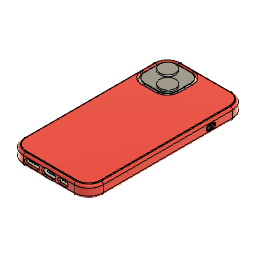
Day 10 - Phone Case v1 (Autodesk Fusion 360 design; units mm, degrees)
Autodesk Fusion 360 part; units mm, degrees
sketch "Sketch1" plane through (0, 0, 0) normal (0, 0, 1) x (1, 0, 0)
  line L0 (-24.135, 73.4) -> (24.135, 73.4)
  line L1 (35.8, 61.735) -> (35.8, -61.735)
  line L2 (24.135, -73.4) -> (-24.135, -73.4)
  line L3 (-35.8, -61.735) -> (-35.8, 61.735)
  arc A0 (-24.135, 73.4) -> (-35.8, 61.735) centre (-24.135, 61.735) ccw
  arc A1 (35.8, 61.735) -> (24.135, 73.4) centre (24.135, 61.735) ccw
  arc A2 (24.135, -73.4) -> (35.8, -61.735) centre (24.135, -61.735) ccw
  arc A3 (-35.8, -61.735) -> (-24.135, -73.4) centre (-24.135, -61.735) ccw
  point P0 (35.8, 73.4)
  point P1 (35.8, -73.4)
  point P2 (-35.8, -73.4)
  dimension "d1" = 71.6
  dimension "d2" = 146.8
  dimension "d3" = 11.665
  constraint horizontal L0
  constraint perpendicular L0 L1
  constraint parallel L0 L2
  constraint parallel L1 L3
  constraint tangent L0 A0
  constraint tangent L3 A0
  constraint coincident P0 L0
  constraint coincident P0 L1
  constraint tangent L0 A1
  constraint tangent L1 A1
  constraint equal A0 A1
  constraint coincident P1 L1
  constraint coincident P1 L2
  constraint tangent L1 A2
  constraint tangent L2 A2
  constraint equal A0 A2
  constraint coincident P2 L2
  constraint coincident P2 L3
  constraint tangent L2 A3
  constraint tangent L3 A3
  constraint equal A0 A3
  measures "d1" distance of P1 P2
  measures "d2" distance of P0 P1
  measures "d3" radius of A0
extrude "Extrude1" add sketch "Sketch1" along normal blind 7.8 makes body 1
fillet "Fillet1" radius 0.4 2 faces at (-11.9333, 20.5783, 7.8) (-11.9333, 20.5783, 0) on bodies 1
sketch "Sketch2" plane through (0, 0, 7.8) normal (0, 0, 1) x (-1, 0, 0)
  arc A0 (24.135, -73) -> (35.4, -61.735) centre (24.135, -61.735) ccw
  line L0 (35.4, -61.735) -> (35.4, 61.735)
  arc A1 (35.4, 61.735) -> (24.135, 73) centre (24.135, 61.735) ccw
  line L1 (24.135, 73) -> (-24.135, 73)
  arc A2 (-24.135, 73) -> (-35.4, 61.735) centre (-24.135, 61.735) ccw
  line L2 (-35.4, 61.735) -> (-35.4, -61.735)
  arc A3 (-35.4, -61.735) -> (-24.135, -73) centre (-24.135, -61.735) ccw
  line L3 (-24.135, -73) -> (24.135, -73)
  arc A4 (24.135, -73.4) -> (35.8, -61.735) centre (24.135, -61.735) ccw
  line L4 (35.8, 61.735) -> (35.8, -61.735)
  arc A5 (35.8, 61.735) -> (24.135, 73.4) centre (24.135, 61.735) ccw
  line L5 (-24.135, 73.4) -> (24.135, 73.4)
  arc A6 (-24.135, 73.4) -> (-35.8, 61.735) centre (-24.135, 61.735) ccw
  line L6 (-35.8, -61.735) -> (-35.8, 61.735)
  arc A7 (-35.8, -61.735) -> (-24.135, -73.4) centre (-24.135, -61.735) ccw
  line L7 (24.135, -73.4) -> (-24.135, -73.4)
  line L8 (21.4109, -73.4) -> (21.4109, -70.7)
  line L9 (35.8, -59.3465) -> (33.1, -59.3465)
  line L10 (24.118, -70.7) -> (11.082, -70.7)
  line L11 (2.1, -61.718) -> (2.1, -48.682)
  line L12 (11.082, -39.7) -> (24.118, -39.7)
  line L13 (33.1, -48.682) -> (33.1, -61.718)
  arc A8 (24.118, -70.7) -> (33.1, -61.718) centre (24.118, -61.718) ccw
  arc A9 (2.1, -61.718) -> (11.082, -70.7) centre (11.082, -61.718) ccw
  arc A10 (11.082, -39.7) -> (2.1, -48.682) centre (11.082, -48.682) ccw
  arc A11 (33.1, -48.682) -> (24.118, -39.7) centre (24.118, -48.682) ccw
  point P0 (33.1, -70.7)
  point P1 (2.1, -70.7)
  point P2 (33.1, -39.7)
  dimension "d8" = 2.7
  dimension "d9" = 2.7
  dimension "d10" = 31
  dimension "d11" = 31
  dimension "d12" = 8.982
  constraint coincident L7 L8.start
  constraint perpendicular L3 L8
  constraint coincident L4 L9.start
  constraint perpendicular L0 L9
  constraint horizontal L10
  constraint vertical L11
  constraint horizontal L12
  constraint vertical L13
  constraint coincident P0 L10
  constraint coincident P0 L13
  constraint tangent L10 A8
  constraint tangent L13 A8
  constraint coincident P1 L10
  constraint coincident P1 L11
  constraint tangent L10 A9
  constraint tangent L11 A9
  constraint equal A8 A9
  constraint tangent L11 A10
  constraint tangent L12 A10
  constraint equal A8 A10
  constraint coincident P2 L12
  constraint coincident P2 L13
  constraint tangent L12 A11
  constraint tangent L13 A11
  constraint equal A8 A11
  measures "d8" distance of L8.start L8.end
  measures "d9" distance of L9.start L9.end
  measures "d10" distance of P0 P1
  measures "d11" distance of P0 P2
  measures "d12" radius of A8
extrude "Extrude2" add sketch "Sketch2" along normal blind 2 contours L10 L11 L12 L13 A8 A9 A10 A11 bodies 1
fillet "Fillet2" radius 1.5 8 edges at (-33.1, 55.2, 7.8) (-30.4692, 68.0692, 7.8) (-17.6, 70.7, 7.8) (-4.7308, 68.0692, 7.8) (-2.1, 55.2, 7.8) (-4.7308, 42.3308, 7.8) (-17.6, 39.7, 7.8) (-30.4692, 42.3308, 7.8) on bodies 1
sketch "Sketch3" plane through (0, 0, 9.8) normal (0, 0, 1) x (-1, 0, 0)
  arc A0 (24.118, -70.7) -> (33.1, -61.718) centre (24.118, -61.718) ccw
  line L0 (33.1, -61.718) -> (33.1, -48.682)
  arc A1 (33.1, -48.682) -> (24.118, -39.7) centre (24.118, -48.682) ccw
  line L1 (24.118, -39.7) -> (11.082, -39.7)
  arc A2 (11.082, -39.7) -> (2.1, -48.682) centre (11.082, -48.682) ccw
  line L2 (2.1, -48.682) -> (2.1, -61.718)
  arc A3 (2.1, -61.718) -> (11.082, -70.7) centre (11.082, -61.718) ccw
  line L3 (11.082, -70.7) -> (24.118, -70.7)
  line L4 (21.9339, -70.7) -> (21.9339, -68.7)
  line L5 (33.1, -60.9415) -> (31.1, -60.9415)
  line L6 (12.075, -70.7) -> (12.075, -56.2)
  line L7 (33.1, -49.3388) -> (18.6, -49.3388)
  line L8 (31.1, -68.7) -> (23.6, -68.7)
  line L9 (31.1, -68.7) -> (31.1, -61.2)
  circle A4 centre (23.6, -61.2) radius 7.5
  line L10 (18.6, -56.2) -> (11.1, -56.2)
  line L11 (18.6, -56.2) -> (18.6, -48.7)
  circle A5 centre (11.082, -48.682) radius 7.518
  dimension "d17" = 2
  dimension "d18" = 2
  dimension "d19" = 14.5
  dimension "d20" = 14.5
  dimension "d21" = 7.5
  dimension "d22" = 7.5
  dimension "d23" = 7.5
  dimension "d24" = 7.5
  constraint coincident L3 L4.start
  constraint perpendicular L3 L4
  constraint coincident L0 L5.start
  constraint perpendicular L0 L5
  constraint coincident L3 L6.start
  constraint perpendicular L3 L6
  constraint coincident L0 L7.start
  constraint perpendicular L0 L7
  constraint parallel L3 L8
  constraint perpendicular L5 L9
  constraint coincident L8.end A4
  constraint tangent L8 A4
  constraint perpendicular L6 L10
  constraint perpendicular L7 L11
  constraint concentric A2 A5
  constraint coincident L11.end A5
  measures "d17" distance of L4.start L4.end
  measures "d18" distance of L5.start L5.end
  measures "d19" distance of L6.start L6.end
  measures "d20" distance of L7.start L7.end
  measures "d21" distance of L8.start L8.end
  measures "d22" distance of L8.start L9.end
  measures "d23" distance of L10.start L10.end
  measures "d24" distance of L10.start L11.end
extrude "Extrude3" add sketch "Sketch3" along normal blind 1.5 contours A4 L10 L11 | A5 picked at (25.4599, -63.0599) bodies 1
delete_face "DeleteFace1" 2 faces at (-18.4033, 56.2, 10.3) (-18.6, 56.0033, 10.3) on bodies 1
sketch "Sketch4" plane through (35.8, 0, 0) normal (1, 0, 0) x (0, 1, 0)
  line L0 (-61.735, 0.4) -> (61.735, 0.4)
  line L1 (61.735, 0.4) -> (61.735, 7.4)
  line L2 (61.735, 7.4) -> (-61.735, 7.4)
  line L3 (-61.735, 7.4) -> (-61.735, 0.4)
  line L4 (68.7, 11.3) -> (53.7, 11.3)
  line L5 (70.7, 9.8) -> (68.7, 9.8)
  line L6 (41.164, 9.8) -> (39.7, 9.8)
  line L7 (53.7, 11.3) -> (41.164, 11.3)
  arc A0 (70.7, 9.3) -> (72.2, 7.8) centre (72.2, 9.3) ccw
  arc A1 (38.2, 7.8) -> (39.7, 9.3) centre (38.2, 9.3) ccw
  line L8 (70.7, 9.3) -> (70.7, 9.8)
  line L9 (72.2, 7.8) -> (73, 7.8)
  line L10 (-61.735, 7.8) -> (38.2, 7.8)
  line L11 (-73, 7.8) -> (-61.735, 7.8)
  line L12 (39.7, 9.3) -> (39.7, 9.8)
  arc A2 (73, 0) -> (73.4, 0.4) centre (73, 0.4) ccw
  line L13 (73, 0) -> (61.735, 0)
  line L14 (61.735, 0) -> (-61.735, 0)
  arc A3 (-73.4, 0.4) -> (-73, 0) centre (-73, 0.4) ccw
  line L15 (-61.735, 0) -> (-73, 0)
  line L16 (73.4, 0.4) -> (73.4, 7.4)
  arc A4 (73.4, 7.4) -> (73, 7.8) centre (73, 7.4) ccw
  arc A5 (-73, 7.8) -> (-73.4, 7.4) centre (-73, 7.4) ccw
  line L17 (-73.4, 0.4) -> (-73.4, 7.4)
  line L18 (41.164, 9.8) -> (41.164, 11.3)
  line L19 (68.7, 9.8) -> (68.7, 11.3)
  line L20 (73.4, 3.9) -> (44.07, 3.9)
  line L21 (44.07, 3.9) -> (41.27, 3.9)
  line L22 (43.5325, 4.975) -> (39.0075, 4.975)
  line L23 (38.47, 4.4375) -> (38.47, 3.3625)
  line L24 (39.0075, 2.825) -> (43.5325, 2.825)
  line L25 (44.07, 3.3625) -> (44.07, 4.4375)
  arc A6 (44.07, 4.4375) -> (43.5325, 4.975) centre (43.5325, 4.4375) ccw
  arc A7 (43.5325, 2.825) -> (44.07, 3.3625) centre (43.5325, 3.3625) ccw
  arc A8 (38.47, 3.3625) -> (39.0075, 2.825) centre (39.0075, 3.3625) ccw
  arc A9 (39.0075, 4.975) -> (38.47, 4.4375) centre (39.0075, 4.4375) ccw
  line L26 (38.47, 4.975) -> (44.07, 4.975)
  line L27 (44.07, 4.975) -> (44.07, 4.437)
  line L28 (43.533, 3.9) -> (39.007, 3.9)
  line L29 (38.47, 4.437) -> (38.47, 4.975)
  arc A10 (38.47, 4.437) -> (39.007, 3.9) centre (39.007, 4.437) ccw
  arc A11 (43.533, 3.9) -> (44.07, 4.437) centre (43.533, 4.437) ccw
  line L30 (38.47, 3.9) -> (33.35, 3.9)
  line L31 (33.35, 3.9) -> (22.15, 3.9)
  line L32 (22.15, 3.9) -> (19.05, 3.9)
  line L33 (19.05, 3.9) -> (7.85, 3.9)
  line L34 (23.5, 5.25) -> (32, 5.25)
  line L35 (32, 2.55) -> (23.5, 2.55)
  line L36 (17.7, 2.55) -> (9.2, 2.55)
  line L37 (9.2, 5.25) -> (17.7, 5.25)
  arc A12 (9.2, 5.25) -> (7.85, 3.9) centre (9.2, 3.9) ccw
  arc A13 (7.85, 3.9) -> (9.2, 2.55) centre (9.2, 3.9) ccw
  arc A14 (19.05, 3.9) -> (17.7, 5.25) centre (17.7, 3.9) ccw
  arc A15 (17.7, 2.55) -> (19.05, 3.9) centre (17.7, 3.9) ccw
  arc A16 (23.5, 5.25) -> (22.15, 3.9) centre (23.5, 3.9) ccw
  arc A17 (22.15, 3.9) -> (23.5, 2.55) centre (23.5, 3.9) ccw
  arc A18 (33.35, 3.9) -> (32, 5.25) centre (32, 3.9) ccw
  arc A19 (32, 2.55) -> (33.35, 3.9) centre (32, 3.9) ccw
  point P0 (38.47, 4.975)
  point P1 (38.47, 2.825)
  point P2 (44.07, 2.825)
  point P3 (41.27, 3.9)
  point P4 (33.35, 5.25)
  point P5 (33.35, 2.55)
  point P6 (27.75, 3.9)
  point P7 (7.85, 2.55)
  point P8 (7.85, 5.25)
  point P9 (13.45, 3.9)
  dimension "d27" = 29.33
  dimension "d29" = 2.8
  dimension "d30" = 5.6
  dimension "d31" = 2.15
  dimension "d32" = 0.5375
  dimension "d33" = 0.537
  dimension "d34" = 5.12
  dimension "d35" = 11.2
  dimension "d36" = 3.1
  dimension "d37" = 11.2
  dimension "d38" = 2.7
  dimension "d39" = 2.7
  dimension "d40" = 1.35
  dimension "d41" = 1.35
  dimension "d42" = 1.35
  dimension "d43" = 1.35
  dimension "d44" = 1.35
  dimension "d45" = 1.35
  dimension "d46" = 1.35
  dimension "d47" = 1.35
  constraint midpoint L16 L20.start
  constraint perpendicular L1 L20
  constraint perpendicular L18 L21
  constraint horizontal L22
  constraint perpendicular L22 L23
  constraint parallel L22 L24
  constraint parallel L23 L25
  constraint coincident P3 L21.end
  constraint tangent L22 A6
  constraint tangent L25 A6
  constraint coincident P2 L24
  constraint coincident P2 L25
  constraint tangent L24 A7
  constraint tangent L25 A7
  constraint equal A6 A7
  constraint coincident P1 L23
  constraint coincident P1 L24
  constraint tangent L23 A8
  constraint tangent L24 A8
  constraint equal A6 A8
  constraint coincident P0 L22
  constraint coincident P0 L23
  constraint tangent L22 A9
  constraint tangent L23 A9
  constraint equal A6 A9
  constraint horizontal L26
  constraint vertical L27
  constraint horizontal L28
  constraint vertical L29
  constraint coincident P0 L26.start
  constraint tangent L28 A10
  constraint tangent L29 A10
  constraint coincident L20.end L27
  constraint coincident L20.end L28
  constraint tangent L27 A11
  constraint tangent L28 A11
  constraint equal A10 A11
  constraint midpoint L23 L30.start
  constraint perpendicular L23 L30
  constraint parallel L2 L31
  constraint parallel L31 L32
  constraint parallel L32 L33
  constraint horizontal L34
  constraint parallel L34 L35
  constraint midpoint L31 P6
  constraint horizontal L36
  constraint parallel L36 L37
  constraint midpoint L33 P9
  constraint coincident P8 L37
  constraint tangent L37 A12
  constraint coincident P7 L36
  constraint tangent L36 A13
  constraint coincident L33.end A12.end
  constraint tangent L37 A14
  constraint tangent L36 A15
  constraint coincident L32.end L33.start
  constraint tangent L34 A16
  constraint tangent L35 A17
  constraint coincident L31.end L32.start
  constraint coincident P4 L34
  constraint tangent L34 A18
  constraint coincident P5 L35
  constraint tangent L35 A19
  constraint coincident L30.end L31.start
  measures "d27" distance of L20.start L20.end
  measures "d29" distance of L20.end P3
  measures "d30" distance of P1 P2
  measures "d31" distance of P0 P1
  measures "d32" radius of A6
  measures "d33" radius of A10
  measures "d34" distance of L30.start L30.end
  measures "d35" distance of L30.end L31.end
  measures "d36" distance of L31.end L32.end
  measures "d37" distance of L32.end L33.end
  measures "d38" distance of P4 P5
  measures "d39" distance of P7 P8
  measures "d40" radius of A12
  measures "d41" radius of A13
  measures "d42" radius of A14
  measures "d43" radius of A15
  measures "d44" radius of A16
  measures "d45" radius of A17
  measures "d46" radius of A18
  measures "d47" radius of A19
extrude "Extrude4" add sketch "Sketch4" along normal blind 0.6 contours L21 L22 A6 A9 L26 L28 A10 A11 | L31 L35 A17 A19 | L31 L34 A16 A18 | L33 L36 A13 A15 | L33 L37 A12 A14 bodies 1
extrude "Extrude5" cut sketch "Sketch4" against normal blind 0.6 contours L21 L23 L24 L25 A7 A8 L28 A10 A11 bodies 1
sketch "Sketch5" plane through (-35.8, 0, 0) normal (-1, 0, 0) x (0, -1, 0)
  line L0 (-61.735, 0.4) -> (61.735, 0.4)
  line L1 (61.735, 0.4) -> (61.735, 7.4)
  line L2 (61.735, 7.4) -> (-61.735, 7.4)
  line L3 (-61.735, 7.4) -> (-61.735, 0.4)
  line L4 (-63.1098, 11.3) -> (-68.7, 11.3)
  line L5 (-56.2, 11.3) -> (-63.1098, 11.3)
  line L6 (-39.7, 9.8) -> (-41.164, 9.8)
  line L7 (-68.7, 9.8) -> (-70.7, 9.8)
  line L8 (-48.682, 11.3) -> (-56.2, 11.3)
  line L9 (-41.164, 11.3) -> (-48.682, 11.3)
  arc A0 (-72.2, 7.8) -> (-70.7, 9.3) centre (-72.2, 9.3) ccw
  arc A1 (-39.7, 9.3) -> (-38.2, 7.8) centre (-38.2, 9.3) ccw
  line L10 (-70.7, 9.3) -> (-70.7, 9.8)
  line L11 (61.735, 7.8) -> (73, 7.8)
  line L12 (-38.2, 7.8) -> (61.735, 7.8)
  line L13 (-73, 7.8) -> (-72.2, 7.8)
  line L14 (-39.7, 9.3) -> (-39.7, 9.8)
  arc A2 (73, 0) -> (73.4, 0.4) centre (73, 0.4) ccw
  line L15 (73, 0) -> (61.735, 0)
  line L16 (61.735, 0) -> (-61.735, 0)
  arc A3 (-73.4, 0.4) -> (-73, 0) centre (-73, 0.4) ccw
  line L17 (-61.735, 0) -> (-73, 0)
  line L18 (-73.4, 0.4) -> (-73.4, 7.4)
  arc A4 (73.4, 7.4) -> (73, 7.8) centre (73, 7.4) ccw
  arc A5 (-73, 7.8) -> (-73.4, 7.4) centre (-73, 7.4) ccw
  line L19 (73.4, 0.4) -> (73.4, 7.4)
  line L20 (-41.164, 9.8) -> (-41.164, 11.3)
  line L21 (-68.7, 9.8) -> (-68.7, 11.3)
  line L22 (-73.4, 3.9) -> (-29.5, 3.9)
  line L23 (-29.5, 3.9) -> (-11.8, 3.9)
  line L24 (-13.15, 5.25) -> (-28.15, 5.25)
  line L25 (-29.5, 3.9) -> (-29.5, 4)
  line L26 (-28.05, 2.55) -> (-13.15, 2.55)
  arc A6 (-28.15, 5.25) -> (-29.5, 3.9) centre (-28.15, 3.9) ccw
  arc A7 (-29.5, 4) -> (-28.05, 2.55) centre (-28.05, 4) ccw
  arc A8 (-11.8, 3.9) -> (-13.15, 5.25) centre (-13.15, 3.9) ccw
  arc A9 (-13.15, 2.55) -> (-11.8, 3.9) centre (-13.15, 3.9) ccw
  point P0 (-29.5, 5.25)
  point P1 (-29.5, 2.55)
  point P2 (-20.65, 3.9)
  dimension "d52" = 43.9
  dimension "d53" = 17.7
  dimension "d54" = 2.7
  dimension "d55" = 1.35
  dimension "d56" = 1.45
  dimension "d57" = 1.35
  dimension "d58" = 1.35
  constraint midpoint L18 L22.start
  constraint perpendicular L18 L22
  constraint parallel L22 L23
  constraint horizontal L24
  constraint perpendicular L24 L25
  constraint parallel L24 L26
  constraint midpoint L23 P2
  constraint coincident P0 L24
  constraint coincident P0 L25
  constraint tangent L24 A6
  constraint tangent L25 A6
  constraint coincident P1 L25
  constraint coincident P1 L26
  constraint tangent L25 A7
  constraint tangent L26 A7
  constraint tangent L24 A8
  constraint tangent L26 A9
  constraint coincident L23.end A8.start
  measures "d52" distance of L22.start L22.end
  measures "d53" distance of L22.end L23.end
  measures "d54" distance of P0 P1
  measures "d55" radius of A6
  measures "d56" radius of A7
  measures "d57" radius of A8
  measures "d58" radius of A9
extrude "Extrude6" add sketch "Sketch5" along normal blind 0.6 contours L23 L24 L25 A6 A7 A8 | L23 L26 A7 A9 bodies 1
sketch "Sketch6" plane through (0, -73.4, 0) normal (0, -1, 0) x (1, 0, 0)
  line L0 (-24.135, 0.4) -> (24.135, 0.4)
  line L1 (24.135, 0.4) -> (24.135, 7.4)
  line L2 (24.135, 7.4) -> (-24.135, 7.4)
  line L3 (-24.135, 7.4) -> (-24.135, 0.4)
  line L4 (-35.8, 2.55) -> (-36.4, 2.55)
  line L5 (-36.4, 3.9491) -> (-36.4, 2.55)
  line L6 (-36.4, 5.25) -> (-36.4, 3.9491)
  line L7 (-35.8, 5.25) -> (-36.4, 5.25)
  line L8 (35.8, 5.25) -> (36.4, 5.25)
  line L9 (36.4, 2.55) -> (36.4, 3.9)
  line L10 (36.4, 4.975) -> (36.4, 5.25)
  line L11 (35.8, 2.55) -> (36.4, 2.55)
  line L12 (36.4, 4.4375) -> (36.4, 4.975)
  line L13 (36.4, 4.437) -> (36.4, 4.4375)
  line L14 (36.4, 3.9) -> (36.4, 4.437)
  line L15 (-16.3472, 11.3) -> (-31.1, 11.3)
  line L16 (-16.1, 11.3) -> (-16.3472, 11.3)
  line L17 (-31.1, 9.8) -> (-33.1, 9.8)
  line L18 (-2.1, 9.8) -> (-3.564, 9.8)
  line L19 (-3.564, 11.3) -> (-16.1, 11.3)
  arc A0 (-34.6, 7.8) -> (-33.1, 9.3) centre (-34.6, 9.3) ccw
  arc A1 (-2.1, 9.3) -> (-0.6, 7.8) centre (-0.6, 9.3) ccw
  line L20 (-2.1, 9.3) -> (-2.1, 9.8)
  line L21 (-33.1, 9.3) -> (-33.1, 9.8)
  line L22 (-35.4, 7.8) -> (-34.6, 7.8)
  line L23 (24.135, 7.8) -> (35.4, 7.8)
  line L24 (-0.6, 7.8) -> (24.135, 7.8)
  line L25 (-24.135, 0) -> (-35.4, 0)
  arc A2 (-35.8, 0.4) -> (-35.4, 0) centre (-35.4, 0.4) ccw
  arc A3 (35.4, 0) -> (35.8, 0.4) centre (35.4, 0.4) ccw
  line L26 (35.4, 0) -> (24.135, 0)
  line L27 (24.135, 0) -> (-24.135, 0)
  line L28 (35.8, 0.4) -> (35.8, 2.55)
  line L29 (35.8, 5.25) -> (35.8, 7.4)
  line L30 (-35.8, 0.4) -> (-35.8, 2.55)
  line L31 (-35.8, 5.25) -> (-35.8, 7.4)
  arc A4 (-35.4, 7.8) -> (-35.8, 7.4) centre (-35.4, 7.4) ccw
  arc A5 (35.8, 7.4) -> (35.4, 7.8) centre (35.4, 7.4) ccw
  line L32 (-3.564, 9.8) -> (-3.564, 11.3)
  line L33 (-31.1, 9.8) -> (-31.1, 11.3)
  line L34 (-35.8, 5.25) -> (-35.8, 2.55)
  circle A6 centre (-11.125, 3.9) radius 0.625
  circle A7 centre (-13.475, 3.9) radius 0.625
  circle A8 centre (-15.825, 3.9) radius 0.625
  circle A9 centre (-18.175, 3.9) radius 0.625
  circle A10 centre (-20.525, 3.9) radius 0.625
  dimension "d62" = 1.25
  dimension "d65" = -9.4
  dimension "d66" = 0
  constraint coincident L7.start L31.start
  constraint coincident L4.start L30.end
  measures "d62" diameter of A6
extrude "Extrude7" cut sketch "Sketch6" against normal blind 0.6 contours A6 | A7 | A8 | A9 | A10 bodies 1
sketch "Sketch7" plane through (0, -73.4, 0) normal (0, -1, 0) x (1, 0, 0)
  circle A0 centre (-15.825, 3.9) radius 0.625
  circle A1 centre (-18.175, 3.9) radius 0.625
  circle A2 centre (-13.475, 3.9) radius 0.625
  circle A3 centre (-20.525, 3.9) radius 0.625
  circle A4 centre (-11.125, 3.9) radius 0.625
  line L0 (-24.135, 0.4) -> (24.135, 0.4)
  line L1 (24.135, 0.4) -> (24.135, 7.4)
  line L2 (24.135, 7.4) -> (-24.135, 7.4)
  line L3 (-24.135, 7.4) -> (-24.135, 0.4)
  line L4 (-35.8, 2.55) -> (-36.4, 2.55)
  line L5 (-36.4, 3.9491) -> (-36.4, 2.55)
  line L6 (-36.4, 5.25) -> (-36.4, 3.9491)
  line L7 (-35.8, 5.25) -> (-36.4, 5.25)
  line L8 (35.8, 5.25) -> (36.4, 5.25)
  line L9 (36.4, 2.55) -> (36.4, 3.9)
  line L10 (36.4, 4.975) -> (36.4, 5.25)
  line L11 (35.8, 2.55) -> (36.4, 2.55)
  line L12 (36.4, 4.4375) -> (36.4, 4.975)
  line L13 (36.4, 4.437) -> (36.4, 4.4375)
  line L14 (36.4, 3.9) -> (36.4, 4.437)
  line L15 (-16.3472, 11.3) -> (-31.1, 11.3)
  line L16 (-16.1, 11.3) -> (-16.3472, 11.3)
  line L17 (-31.1, 9.8) -> (-33.1, 9.8)
  line L18 (-2.1, 9.8) -> (-3.564, 9.8)
  line L19 (-3.564, 11.3) -> (-16.1, 11.3)
  arc A5 (-34.6, 7.8) -> (-33.1, 9.3) centre (-34.6, 9.3) ccw
  arc A6 (-2.1, 9.3) -> (-0.6, 7.8) centre (-0.6, 9.3) ccw
  line L20 (-2.1, 9.3) -> (-2.1, 9.8)
  line L21 (-33.1, 9.3) -> (-33.1, 9.8)
  line L22 (-35.4, 7.8) -> (-34.6, 7.8)
  line L23 (24.135, 7.8) -> (35.4, 7.8)
  line L24 (-0.6, 7.8) -> (24.135, 7.8)
  line L25 (-24.135, 0) -> (-35.4, 0)
  arc A7 (-35.8, 0.4) -> (-35.4, 0) centre (-35.4, 0.4) ccw
  arc A8 (35.4, 0) -> (35.8, 0.4) centre (35.4, 0.4) ccw
  line L26 (35.4, 0) -> (24.135, 0)
  line L27 (24.135, 0) -> (-24.135, 0)
  line L28 (35.8, 0.4) -> (35.8, 2.55)
  line L29 (35.8, 5.25) -> (35.8, 7.4)
  line L30 (-35.8, 0.4) -> (-35.8, 2.55)
  line L31 (-35.8, 5.25) -> (-35.8, 7.4)
  arc A9 (-35.4, 7.8) -> (-35.8, 7.4) centre (-35.4, 7.4) ccw
  arc A10 (35.8, 7.4) -> (35.4, 7.8) centre (35.4, 7.4) ccw
  line L32 (-3.564, 9.8) -> (-3.564, 11.3)
  line L33 (-31.1, 9.8) -> (-31.1, 11.3)
  line L34 (35.8, 5.25) -> (35.8, 2.55)
  line L35 (35.8, 3.9) -> (10.5, 3.9)
  circle A11 centre (11.125, 3.9) radius 0.625
  circle A12 centre (13.475, 3.9) radius 0.625
  circle A13 centre (15.825, 3.9) radius 0.625
  dimension "d69" = 25.3
  dimension "d70" = 1.25
  dimension "d73" = 4.7
  dimension "d74" = 0
  constraint coincident L8.start L29.start
  constraint coincident L11.start L28.end
  constraint midpoint L34 L35.start
  constraint perpendicular L34 L35
  constraint coincident L35.end A11
  measures "d69" distance of L35.start L35.end
  measures "d70" diameter of A11
extrude "Extrude8" cut sketch "Sketch7" against normal blind 0.6 contours L35 A11 | L35 A11 | L35 A13 | L35 A13 | L35 A12 | L35 A12 bodies 1
sketch "Sketch8" plane through (0, -73.4, 0) normal (0, -1, 0) x (1, 0, 0)
  circle A0 centre (11.125, 3.9) radius 0.625
  circle A1 centre (13.475, 3.9) radius 0.625
  circle A2 centre (15.825, 3.9) radius 0.625
  circle A3 centre (-15.825, 3.9) radius 0.625
  circle A4 centre (-18.175, 3.9) radius 0.625
  circle A5 centre (-13.475, 3.9) radius 0.625
  circle A6 centre (-20.525, 3.9) radius 0.625
  circle A7 centre (-11.125, 3.9) radius 0.625
  line L0 (-24.135, 0.4) -> (24.135, 0.4)
  line L1 (24.135, 0.4) -> (24.135, 7.4)
  line L2 (24.135, 7.4) -> (-24.135, 7.4)
  line L3 (-24.135, 7.4) -> (-24.135, 0.4)
  line L4 (0, 7.4) -> (0, 3)
  line L5 (24.135, 3.9) -> (0, 3.9)
  line L6 (-2.9, 3.1) -> (2.9, 3.1)
  line L7 (2.9, 4.7) -> (-2.9, 4.7)
  arc A8 (3.7, 3.9) -> (2.9, 4.7) centre (2.9, 3.9) ccw
  arc A9 (2.9, 3.1) -> (3.7, 3.9) centre (2.9, 3.9) ccw
  arc A10 (-2.9, 4.7) -> (-3.7, 3.9) centre (-2.9, 3.9) ccw
  arc A11 (-3.7, 3.9) -> (-2.9, 3.1) centre (-2.9, 3.9) ccw
  point P0 (3.7, 3.1)
  point P1 (3.7, 4.7)
  point P2 (-3.7, 4.7)
  point P3 (0, 3.9)
  dimension "d77" = 7.4
  dimension "d78" = 1.6
  dimension "d79" = 0.8
  dimension "d80" = 0.8
  dimension "d81" = 0.8
  constraint midpoint L2 L4.start
  constraint perpendicular L2 L4
  constraint midpoint L1 L5.start
  constraint coincident L4 P3
  constraint perpendicular L4 L5
  constraint horizontal L6
  constraint parallel L6 L7
  constraint coincident P3 L5.end
  constraint coincident P1 L7
  constraint tangent L7 A8
  constraint coincident P0 L6
  constraint tangent L6 A9
  constraint coincident A8.start A9.end
  constraint coincident P2 L7
  constraint tangent L7 A10
  constraint equal A9 A10
  constraint tangent L6 A11
  constraint coincident A10.end A11.start
  measures "d77" distance of P1 P2
  measures "d78" distance of P0 P1
  measures "d79" radius of A8
  measures "d80" radius of A9
  measures "d81" radius of A11
extrude "Extrude9" cut sketch "Sketch8" against normal blind 1.2 contours L4 L5 L6 A9 | L4 L5 L7 A8 | L4 L6 L7 A10 A11 bodies 1
copy_body "Body->Comp1" bodies 1 removing the originals makes body 2 in component "Phone"
sketch "Sketch1 (2)" plane through (0, 0, 0) normal (0, 1, 0) x (1, 0, 0) in component "Pone Case"
  arc A0 (35.4, -7.8) -> (35.8, -7.4) centre (35.4, -7.4) ccw
  line L0 (35.8, -0.4) -> (35.8, -7.4)
  arc A1 (35.8, -0.4) -> (35.4, 0) centre (35.4, -0.4) ccw
  arc A2 (35.4, -8.05) -> (36.05, -7.4) centre (35.4, -7.4) ccw
  line L1 (36.05, -0.4) -> (36.05, -7.4)
  arc A3 (36.05, -0.4) -> (35.4, 0.25) centre (35.4, -0.4) ccw
  line L2 (35.4, -8.05) -> (35.4, -9.3)
  line L3 (35.4, -9.3) -> (38.05, -9.3)
  line L4 (38.05, -9.3) -> (38.05, 2.25)
  line L5 (38.05, 2.25) -> (35.4, 2.25)
  line L6 (35.4, 2.25) -> (35.4, 0.25)
  dimension "d84" = 0.25
  dimension "d85" = 1.25
  dimension "d86" = 2
  dimension "d87" = 2
  constraint vertical L2
  constraint perpendicular L2 L3
  constraint perpendicular L3 L4
  constraint perpendicular L4 L5
  constraint perpendicular L5 L6
  constraint coincident A0.start L2
  constraint coincident A1.end L6
  measures "d85" distance of A2.start L2.end
  measures "d86" distance of A3.end L5.end
  measures "d87" distance of L1 L4
sweep "Sweep1" add profiles "Sketch1 (2)" along 8 edges at (0, -73, 7.8) (-32.1006, -69.7006, 7.8) (-35.4, 0, 7.8) (-32.1006, 69.7006, 7.8) (0, 73, 7.8) (32.1006, 69.7006, 7.8) (35.4, 0, 7.8) (32.1006, -69.7006, 7.8) section 1 separate body on bodies 2 makes body 3 in component "Pone Case"
fillet "Fillet1'" radius 2 8 edges at (0, -75.65, 9.3) (-33.9744, -71.5744, 9.3) (-38.05, 0, 9.3) (-33.9744, 71.5744, 9.3) (0, 75.65, 9.3) (33.9744, 71.5744, 9.3) (38.05, 0, 9.3) (33.9744, -71.5744, 9.3) on bodies 3 in component "Pone Case"
fillet "Fillet1'" radius 3 8 edges at (0, -75.65, -2.25) (-33.9744, -71.5744, -2.25) (-38.05, 0, -2.25) (-33.9744, 71.5744, -2.25) (0, 75.65, -2.25) (33.9744, 71.5744, -2.25) (38.05, 0, -2.25) (33.9744, -71.5744, -2.25) on bodies 3 in component "Pone Case"
chamfer "Chamfer1" distance 0.5 angle 45 8 edges at (-35.4, 0, 9.3) (-32.1006, 69.7006, 9.3) (0, 73, 9.3) (32.1006, 69.7006, 9.3) (35.4, 0, 9.3) (32.1006, -69.7006, 9.3) (0, -73, 9.3) (-32.1006, -69.7006, 9.3) on bodies 3 in component "Pone Case"
sketch "Sketch3 (2)" plane through (0, 0, 7.8) normal (0, 0, 1) x (-1, 0, 0) in component "Pone Case"
  arc A0 (24.135, -73) -> (35.4, -61.735) centre (24.135, -61.735) ccw
  line L0 (35.4, -61.735) -> (35.4, 61.735)
  arc A1 (35.4, 61.735) -> (24.135, 73) centre (24.135, 61.735) ccw
  line L1 (24.135, 73) -> (-24.135, 73)
  arc A2 (-24.135, 73) -> (-35.4, 61.735) centre (-24.135, 61.735) ccw
  line L2 (-35.4, 61.735) -> (-35.4, -61.735)
  arc A3 (-35.4, -61.735) -> (-24.135, -73) centre (-24.135, -61.735) ccw
  line L3 (-24.135, -73) -> (24.135, -73)
  line L4 (34.6, -48.682) -> (34.6, -61.718)
  arc A4 (24.118, -72.2) -> (34.6, -61.718) centre (24.118, -61.718) ccw
  line L5 (24.118, -72.2) -> (11.082, -72.2)
  arc A5 (0.6, -61.718) -> (11.082, -72.2) centre (11.082, -61.718) ccw
  line L6 (0.6, -61.718) -> (0.6, -48.682)
  arc A6 (11.082, -38.2) -> (0.6, -48.682) centre (11.082, -48.682) ccw
  line L7 (11.082, -38.2) -> (24.118, -38.2)
  arc A7 (34.6, -48.682) -> (24.118, -38.2) centre (24.118, -48.682) ccw
  arc A8 (24.118, -70.7) -> (33.1, -61.718) centre (24.118, -61.718) ccw
  line L8 (33.1, -61.718) -> (33.1, -48.682)
  arc A9 (33.1, -48.682) -> (24.118, -39.7) centre (24.118, -48.682) ccw
  line L9 (24.118, -39.7) -> (11.082, -39.7)
  arc A10 (11.082, -39.7) -> (2.1, -48.682) centre (11.082, -48.682) ccw
  line L10 (2.1, -48.682) -> (2.1, -61.718)
  arc A11 (2.1, -61.718) -> (11.082, -70.7) centre (11.082, -61.718) ccw
  line L11 (11.082, -70.7) -> (24.118, -70.7)
  circle A12 centre (23.6, -61.2) radius 7.5
  circle A13 centre (11.082, -48.682) radius 7.518
  line L12 (11.082, -71.7) -> (24.118, -71.7)
  arc A14 (24.118, -71.7) -> (34.1, -61.718) centre (24.118, -61.718) ccw
  line L13 (34.1, -61.718) -> (34.1, -48.682)
  arc A15 (34.1, -48.682) -> (24.118, -38.7) centre (24.118, -48.682) ccw
  line L14 (24.118, -38.7) -> (11.082, -38.7)
  arc A16 (11.082, -38.7) -> (1.1, -48.682) centre (11.082, -48.682) ccw
  line L15 (1.1, -48.682) -> (1.1, -61.718)
  arc A17 (1.1, -61.718) -> (11.082, -71.7) centre (11.082, -61.718) ccw
  dimension "d99" = 1
extrude "Extrude1'" add sketch "Sketch3 (2)" along normal blind 2 contours A0 L0 A1 L1 A2 L2 A3 L3 bodies 3 in component "Pone Case"
fillet "Fillet2'" radius 1 8 edges at (-31.5299, 41.2701, 9.8) (-34.6, 55.2, 9.8) (-31.5299, 69.1299, 9.8) (-17.6, 72.2, 9.8) (-3.6701, 69.1299, 9.8) (-0.6, 55.2, 9.8) (-3.6701, 41.2701, 9.8) (-17.6, 38.2, 9.8) on bodies 3 in component "Pone Case"
sketch "Sketch6 (2)" plane through (0, -75.65, 0) normal (0, -1, 0) x (1, 0, 0) in component "Pone Case"
  line L0 (-24.135, 0.7295) -> (24.135, 0.7295)
  line L1 (24.135, 0.7295) -> (24.135, 7.3)
  line L2 (24.135, 7.3) -> (-24.135, 7.3)
  line L3 (-24.135, 7.3) -> (-24.135, 0.7295)
  circle A0 centre (-20.525, 3.9) radius 0.625
  circle A1 centre (-18.175, 3.9) radius 0.625
  circle A2 centre (-15.825, 3.9) radius 0.625
  circle A3 centre (-13.475, 3.9) radius 0.625
  circle A4 centre (-11.125, 3.9) radius 0.625
  arc A5 (-2.9, 4.7) -> (-2.9, 3.1) centre (-2.9, 3.9) ccw
  line L4 (-2.9, 3.1) -> (2.9, 3.1)
  arc A6 (2.9, 3.1) -> (2.9, 4.7) centre (2.9, 3.9) ccw
  line L5 (2.9, 4.7) -> (-2.9, 4.7)
  circle A7 centre (11.125, 3.9) radius 0.625
  circle A8 centre (13.475, 3.9) radius 0.625
  circle A9 centre (13.475, 3.9) radius 0.625
  circle A10 centre (15.825, 3.9) radius 0.625
  arc A11 (15.8267, 3.275) -> (15.8233, 4.525) centre (15.825, 3.9) ccw
  line L6 (15.8233, 4.525) -> (11.125, 4.525)
  arc A12 (11.125, 4.525) -> (11.125, 3.275) centre (11.125, 3.9) ccw
  line L7 (11.125, 3.275) -> (15.8267, 3.275)
  arc A13 (-11.125, 3.275) -> (-11.125, 4.525) centre (-11.125, 3.9) ccw
  arc A14 (-20.525, 4.525) -> (-20.525, 3.275) centre (-20.525, 3.9) ccw
  line L8 (-11.125, 4.525) -> (-20.525, 4.525)
  line L9 (-20.525, 3.275) -> (-11.125, 3.275)
  arc A15 (11.125, 5.525) -> (11.125, 2.275) centre (11.125, 3.9) ccw
  line L10 (11.125, 2.275) -> (15.828, 2.275)
  arc A16 (15.828, 2.275) -> (15.822, 5.525) centre (15.825, 3.9) ccw
  line L11 (15.822, 5.525) -> (11.125, 5.525)
  arc A17 (-11.125, 2.275) -> (-11.125, 5.525) centre (-11.125, 3.9) ccw
  line L12 (-11.125, 5.525) -> (-20.525, 5.525)
  arc A18 (-20.525, 5.525) -> (-20.525, 2.275) centre (-20.525, 3.9) ccw
  line L13 (-20.525, 2.275) -> (-11.125, 2.275)
  dimension "d110" = 1
  dimension "d111" = 1
  constraint coincident A10 A11.end
  constraint coincident A10 A11.start
  constraint coincident A10.centre A11.centre
  constraint coincident A7 L6.end
  constraint tangent A7 L6
  constraint horizontal L6
  constraint coincident A7 A12.end
  constraint coincident A7.centre A12.centre
  constraint coincident A4 A13.end
  constraint coincident A4 A13.start
  constraint coincident A4.centre A13.centre
  constraint coincident A0 A14.end
  constraint coincident A0 A14.start
  constraint coincident A0.centre A14.centre
  constraint tangent A0 L8
  constraint tangent A13 L9
extrude "Extrude2'" cut sketch "Sketch6 (2)" against normal up to surface (2 mm away) contours A0 A14 | A0 A1 L8 L9 | A1 A2 L8 L9 | A1 | A2 A3 L8 L9 | A2 | A3 A4 L8 L9 | A3 | A4 A13 | A5 L4 A6 L5 | A7 A12 | A7 A8 A9 L6 L7 | A8 A9 A10 L6 L7 | A8 A9 | A15 L10 A16 L11 | A17 L12 A18 L13 bodies 3 in component "Pone Case"
move_face "OffsetFaces1" offset -2 4 faces at (0.9667, -74.9833, 4.7) (3.3171, -74.3167, 4.5826) (-3.3171, -74.3167, 3.2174) (-0.9667, -74.9833, 3.1) on bodies 3 in component "Pone Case"
chamfer "Chamfer2" distance 1 angle 45 4 edges at (0, -75.65, 1.1) (-5.7, -75.65, 3.9) (0, -75.65, 6.7) (5.7, -75.65, 3.9) on bodies 3 in component "Pone Case"
chamfer "Chamfer2" distance 1 angle 45 8 edges at (17.45, -75.65, 3.903) (13.4735, -75.65, 5.525) (13.4765, -75.65, 2.275) (9.5, -75.65, 3.9) (-9.5, -75.65, 3.9) (-15.825, -75.65, 2.275) (-22.15, -75.65, 3.9) (-15.825, -75.65, 5.525) on bodies 3 in component "Pone Case"
chamfer "Chamfer2" distance 1 angle 45 8 edges at (-15.825, -73.65, 2.275) (-9.5, -73.65, 3.9) (-15.825, -73.65, 5.525) (-22.15, -73.65, 3.9) (13.4765, -73.65, 2.275) (13.4735, -73.65, 5.525) (9.5, -73.65, 3.9) (17.45, -73.65, 3.903) on bodies 3 in component "Pone Case"
chamfer "Chamfer3" distance 1 angle 45 4 edges at (0, -73.65, 1.1) (5.7, -73.65, 3.9) (0, -73.65, 6.7) (-5.7, -73.65, 3.9) on bodies 3 in component "Pone Case"
fillet "Fillet3" radius 1 8 edges at (-17.6, 38.2, 7.8) (-31.5299, 41.2701, 7.8) (-34.6, 55.2, 7.8) (-31.5299, 69.1299, 7.8) (-17.6, 72.2, 7.8) (-3.6701, 69.1299, 7.8) (-0.6, 55.2, 7.8) (-3.6701, 41.2701, 7.8) on bodies 3 in component "Pone Case"
sketch "Sketch12" plane through (38.05, 0, 0) normal (1, 0, 0) x (0, 1, 0) in component "Pone Case"
  line L0 (-61.735, 0.7295) -> (61.735, 0.7295)
  line L1 (61.735, 0.7295) -> (61.735, 7.3)
  line L2 (61.735, 7.3) -> (-61.735, 7.3)
  line L3 (-61.735, 7.3) -> (-61.735, 0.7295)
  line L4 (38.47, 4.4375) -> (38.47, 4.437)
  arc A0 (38.47, 4.437) -> (39.007, 3.9) centre (39.007, 4.437) ccw
  line L5 (39.007, 3.9) -> (43.533, 3.9)
  arc A1 (43.533, 3.9) -> (44.07, 4.437) centre (43.533, 4.437) ccw
  line L6 (44.07, 4.437) -> (44.07, 4.4375)
  arc A2 (44.07, 4.4375) -> (43.5325, 4.975) centre (43.5325, 4.4375) ccw
  line L7 (43.5325, 4.975) -> (39.0075, 4.975)
  arc A3 (39.0075, 4.975) -> (38.47, 4.4375) centre (39.0075, 4.4375) ccw
  line L8 (44.07, 3.3625) -> (44.07, 4.437)
  arc A4 (43.533, 3.9) -> (44.07, 4.437) centre (43.533, 4.437) ccw
  line L9 (43.533, 3.9) -> (39.007, 3.9)
  arc A5 (38.47, 4.437) -> (39.007, 3.9) centre (39.007, 4.437) ccw
  line L10 (38.47, 4.437) -> (38.47, 3.3625)
  arc A6 (38.47, 3.3625) -> (39.0075, 2.825) centre (39.0075, 3.3625) ccw
  line L11 (39.0075, 2.825) -> (43.5325, 2.825)
  arc A7 (43.5325, 2.825) -> (44.07, 3.3625) centre (43.5325, 3.3625) ccw
  line L12 (39.0075, 4.975) -> (43.5325, 4.975)
  line L13 (44.07, 4.4375) -> (44.07, 3.3625)
  line L14 (43.5325, 2.825) -> (39.0075, 2.825)
  line L15 (38.47, 3.3625) -> (38.47, 4.437)
  arc A8 (39.0075, 4.975) -> (38.47, 4.437) centre (39.0075, 4.4375) ccw
  arc A9 (44.07, 4.4375) -> (43.5325, 4.975) centre (43.5325, 4.4375) ccw
  arc A10 (43.5325, 2.825) -> (44.07, 3.3625) centre (43.5325, 3.3625) ccw
  arc A11 (38.47, 3.3625) -> (39.0075, 2.825) centre (39.0075, 3.3625) ccw
  arc A12 (45.07, 4.4375) -> (43.5325, 5.975) centre (43.5325, 4.4375) ccw
  line L16 (39.0075, 5.975) -> (43.5325, 5.975)
  arc A13 (39.0075, 5.975) -> (37.47, 4.4365) centre (39.0075, 4.4375) ccw
  line L17 (37.47, 3.3625) -> (37.47, 4.4365)
  arc A14 (37.47, 3.3625) -> (39.0075, 1.825) centre (39.0075, 3.3625) ccw
  line L18 (43.5325, 1.825) -> (39.0075, 1.825)
  arc A15 (43.5325, 1.825) -> (45.07, 3.3625) centre (43.5325, 3.3625) ccw
  line L19 (45.07, 4.4375) -> (45.07, 3.3625)
  dimension "d118" = 1
  constraint coincident L7.end A3.start
  constraint coincident A2.end L7.start
  constraint coincident L6.end A2.start
  constraint coincident L8.start A7.end
  constraint coincident L11.end A7.start
  constraint coincident A6.end L11.start
  constraint coincident L10.end A6.start
  constraint coincident L4.end A0.start
extrude "Extrude3'" cut sketch "Sketch12" against normal up to surface (2 mm away) contours A0 L5 A1 A2 L7 A3 A4 L9 A5 L12 A8 A9 | A0 L5 A1 L8 A4 L9 A5 L10 A6 L11 A7 L13 L14 L15 A10 A11 | A12 L16 A13 L17 A14 L18 A15 L19 bodies 3 in component "Pone Case"
fillet "Fillet4" radius 0.5 8 edges at (38.05, 37.47, 3.8995) (38.05, 37.92, 5.5243) (38.05, 41.27, 5.975) (38.05, 44.6197, 5.5247) (38.05, 45.07, 3.9) (38.05, 44.6197, 2.2753) (38.05, 41.27, 1.825) (38.05, 37.9203, 2.2753) on bodies 3 in component "Pone Case"
fillet "Fillet4" radius 0.5 8 edges at (36.05, 45.07, 3.9) (36.05, 44.6197, 5.5247) (36.05, 41.27, 5.975) (36.05, 37.92, 5.5243) (36.05, 37.47, 3.8995) (36.05, 37.9203, 2.2753) (36.05, 41.27, 1.825) (36.05, 44.6197, 2.2753) on bodies 3 in component "Pone Case"
component "Phone" placed x (1, 0, 0) y (0, 1, 0) z (0, 0, 1) at (0, 0, 0)
component "Pone Case" placed x (1, 0, 0) y (0, 1, 0) z (0, 0, 1) at (0, 0, 0)
named bodies: "Phone"
